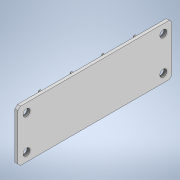
# Autodesk Inventor part: Halterung Gläser1,0
Saved by Autodesk Inventor 2021.3 (Build 253353000, 353)
## iProperties
Created: 2021-10-11
Part Number: Halterung Gläser1,0
Material: Generisch
Document SubType Name: Modeling
Designer: bhelg
Density: 1 g/cm^3
Appearance: Vorgabe
Author: bhelg
Autodesk Inventor part; units mm, degrees
ref_plane "YZ Plane" through (0, 0, 0) normal (1, 0, 0) x (0, 1, 0)
ref_plane "XZ Plane" through (0, 0, 0) normal (0, 1, 0) x (-1, 0, 0)
ref_plane "XY Plane" through (0, 0, 0) normal (0, 0, 1) x (1, 0, 0)
sketch "Skizze1" plane through (0, 0, 0) normal (0, 1, 0) x (-1, 0, 0)
  line L0 (10.8901, 21.3821) -> (14.3901, 21.3821)
  line L1 (14.3901, 21.3821) -> (14.3901, -158.6179)
  line L2 (14.3901, -158.6179) -> (10.8901, -158.6179)
  line L3 (10.8901, -158.6179) -> (10.8901, 21.3821)
  dimension "d0" = 180
  dimension "d1" = 3.5
  constraints: 8 end point, 3 perpendicular, 1 horizontal
  measures "d0" distance of L0.end L1.end
  measures "d1" distance of L0.start L0.end
extrude "Extrusion1" add sketch "Skizze1" along normal blind 60
sketch "Skizze2" plane through (-14.3901, 0, -158.6179) normal (-1, 0, 0) x (0, 0, 1)
  line L0 (0, 0) -> (180, 0) projected
  circle A0 centre (33, 16.5) radius 8.3 construction
  circle A1 centre (33, 43.5) radius 8.3 construction
  circle A2 centre (90, 30) radius 72.5 construction
  line L1 (0, 0) -> (0, 60) projected
  line L2 (0, 60) -> (180, 60) projected
  circle A3 centre (71, 16.5) radius 8.3 construction
  circle A4 centre (109, 16.5) radius 8.3 construction
  circle A5 centre (147, 16.5) radius 8.3 construction
  circle A6 centre (72.7786, 43.5) radius 8.3 construction
  circle A7 centre (109.0755, 43.5) radius 8.3 construction
  circle A8 centre (144.3092, 43.5) radius 8.3 construction
  circle A9 centre (33, 16.5) radius 9.8
  circle A10 centre (23.2, 16.5) radius 1.5
  circle A11 centre (33, 26.3) radius 1.5
  circle A12 centre (42.8, 16.5) radius 1.5
  circle A13 centre (33, 6.7) radius 1.5
  circle A14 centre (33, 43.5) radius 9.8
  circle A15 centre (23.2, 43.5) radius 1.5
  circle A16 centre (33, 53.3) radius 1.5
  circle A17 centre (42.8, 43.5) radius 1.5
  circle A18 centre (33, 33.7) radius 1.5
  point P0 (158.6179, 0)
  dimension "d38" = 16.6
  dimension "d39" = 16.6
  dimension "d42" = 145
  dimension "d43" = 90
  dimension "d44" = 30
  dimension "d50" = 33
  dimension "d51" = 33
  dimension "d52" = 16.5
  dimension "d53" = 16.5
  dimension "d63" = 16.6
  dimension "d64" = 16.6
  dimension "d65" = 16.6
  dimension "d66" = 16.6
  dimension "d67" = 16.6
  dimension "d68" = 16.6
  dimension "d69" = 38
  dimension "d70" = 38
  dimension "d71" = 38
  dimension "d98" = 19.6
  dimension "d99" = 3
  dimension "d100" = 3
  dimension "d101" = 3
  dimension "d102" = 3
  dimension "d103" = 19.6
  dimension "d104" = 3
  dimension "d105" = 3
  dimension "d106" = 3
  dimension "d107" = 3
  constraints: 19 centre point, 8 point on circle, 2 coincident
  measures "d38" diameter of A0
  measures "d39" diameter of A1
  measures "d42" diameter of A2
  measures "d43" horizontal distance of A2.centre L0.start
  measures "d44" vertical distance of L0.start A2.centre
  measures "d50" distance from line of L1 A0.centre
  measures "d51" distance from line of L1 A1.centre
  measures "d52" distance from line of L0 A0.centre
  measures "d53" distance from line of L2 A1.centre
  measures "d63" diameter of A3
  measures "d64" diameter of A4
  measures "d65" diameter of A5
  measures "d66" diameter of A6
  measures "d67" diameter of A7
  measures "d68" diameter of A8
  measures "d69" distance of A3.centre A0.centre
  measures "d70" distance of A4.centre A3.centre
  measures "d71" distance of A4.centre A5.centre
  measures "d98" diameter of A9
  measures "d99" diameter of A10
  measures "d100" diameter of A11
  measures "d101" diameter of A12
  measures "d102" diameter of A13
  measures "d103" diameter of A14
  measures "d104" diameter of A15
  measures "d105" diameter of A16
  measures "d106" diameter of A17
  measures "d107" diameter of A18
sketch "Skizze3" plane through (-14.3901, 0, -158.6179) normal (-1, 0, 0) x (0, 0, 1)
  line L0 (0, 0) -> (180, 0) projected
  line L1 (0, 60) -> (180, 60) projected
  line L2 (180, 0) -> (180, 60) projected
  line L3 (0, 0) -> (0, 60) projected
  line L4 (10, 10) -> (10, 50)
  point P0 (170, 10)
  point P1 (170, 50)
  dimension "d83" = 40
  dimension "d84" = 40
  dimension "d85" = 10
  dimension "d86" = 10
  dimension "d87" = 10
  dimension "d88" = 10
  dimension "d89" = 10
  dimension "d90" = 10
  dimension "d152" = 160
  constraints: 2 end point, 1 vertical
  measures "d83" distance of L4.end L4.start
  measures "d84" distance of point (170, 50) point (170, 10)
  measures "d85" distance from line of L0 point (170, 10)
  measures "d86" distance from line of L1 point (170, 50)
  measures "d87" distance from line of L0 L4.start
  measures "d88" distance from line of L1 L4.end
  measures "d89" distance from line of L2 point (170, 10)
  measures "d90" distance from line of L3 L4.start
  measures "d152" distance of point (170, 10) L4.start
hole "Bohrung1" at (-14.3901, 10, -148.6179) at (-14.3901, 50, -148.6179) at (-14.3901, 10, 11.3821) at (-14.3901, 50, 11.3821) direction (1, 0, 0) diameter 8.2 end through all
extrude "Extrusion3" add sketch "Skizze2" along normal blind 8 contours A9 A12 | A9 A12 | A11 A9 | A9 A11 | A13 A9 | A9 A13 | A10 A9 | A9 A10 | A14 A17 | A14 A17 | A16 A14 | A14 A16 | A18 A14 | A14 A18 | A15 A14 | A14 A15
pattern_linear "Rechteckige Anordnung2" count 4 spacing 37 along (0, 0, 1) of "Extrusion3"
fillet "Rundung1" radius 1 32 edges at (-22.3901, 6.7, -127.1179) (-22.3901, 16.5, -136.9179) (-22.3901, 16.5, -117.3179) (-22.3901, 26.3, -127.1179) (-22.3901, 33.7, -127.1179) (-22.3901, 43.5, -136.9179) (-22.3901, 43.5, -117.3179) (-22.3901, 53.3, -127.1179) (-22.3901, 16.5, -99.9179) (-22.3901, 6.7, -90.1179) (-22.3901, 26.3, -90.1179) (-22.3901, 33.7, -90.1179) (-22.3901, 43.5, -99.9179) (-22.3901, 16.5, -80.3179) (-22.3901, 53.3, -90.1179) (-22.3901, 43.5, -80.3179) (-22.3901, 43.5, -62.9179) (-22.3901, 33.7, -53.1179) (-22.3901, 26.3, -53.1179) (-22.3901, 16.5, -62.9179) (-22.3901, 6.7, -53.1179) (-22.3901, 16.5, -43.3179) (-22.3901, 16.5, -25.9179) (-22.3901, 6.7, -16.1179) (-22.3901, 16.5, -6.3179) (-22.3901, 26.3, -16.1179) (-22.3901, 33.7, -16.1179) (-22.3901, 43.5, -25.9179) (-22.3901, 43.5, -43.3179) (-22.3901, 53.3, -53.1179) (-22.3901, 53.3, -16.1179) (-22.3901, 43.5, -6.3179)
sketch "Skizze4" plane through (-14.3901, 0, -158.6179) normal (-1, 0, 0) x (0, 0, 1)
  line L0 (0, 0) -> (180, 0)
  circle A0 centre (33, 16.5) radius 8.3 construction
  circle A1 centre (33, 43.5) radius 8.3 construction
  circle A2 centre (90, 30) radius 72.5 construction
  line L1 (0, 0) -> (0, 60)
  line L2 (0, 60) -> (180, 60)
  circle A3 centre (71, 16.5) radius 8.3 construction
  circle A4 centre (109, 16.5) radius 8.3 construction
  circle A5 centre (147, 16.5) radius 8.3 construction
  circle A6 centre (72.7786, 43.5) radius 8.3 construction
  circle A7 centre (109.0755, 43.5) radius 8.3 construction
  circle A8 centre (144.3092, 43.5) radius 8.3 construction
  circle A9 centre (33, 16.5) radius 9.8
  circle A10 centre (23.2, 16.5) radius 1.5
  circle A11 centre (33, 26.3) radius 1.5
  circle A12 centre (42.8, 16.5) radius 1.5
  circle A13 centre (33, 6.7) radius 1.5
  circle A14 centre (33, 43.5) radius 9.8
  circle A15 centre (23.2, 43.5) radius 1.5
  circle A16 centre (33, 53.3) radius 1.5
  circle A17 centre (42.8, 43.5) radius 1.5
  circle A18 centre (33, 33.7) radius 1.5
  circle A19 centre (33, 16.5) radius 10.3
  circle A20 centre (33, 43.5) radius 10.3
  point P0 (158.6179, 0)
  point P1 (158.6179, 0)
  point P2 (31.5538, 53.698)
  point P3 (22.802, 44.9462)
  point P4 (23.3148, 44.9956)
  point P5 (31.5044, 53.1852)
  point P6 (22.802, 42.0538)
  point P7 (31.5538, 33.302)
  point P8 (31.5044, 33.8148)
  point P9 (23.3148, 42.0044)
  point P10 (34.4462, 33.302)
  point P11 (43.198, 42.0538)
  point P12 (42.6852, 42.0044)
  point P13 (34.4956, 33.8148)
  point P14 (43.198, 44.9462)
  point P15 (34.4462, 53.698)
  point P16 (34.4956, 53.1852)
  point P17 (42.6852, 44.9956)
  point P18 (31.5538, 26.698)
  point P19 (22.802, 17.9462)
  point P20 (23.3148, 17.9956)
  point P21 (31.5044, 26.1852)
  point P22 (22.802, 15.0538)
  point P23 (31.5538, 6.302)
  point P24 (31.5044, 6.8148)
  point P25 (23.3148, 15.0044)
  point P26 (43.198, 17.9462)
  point P27 (34.4462, 26.698)
  point P28 (34.4956, 26.1852)
  point P29 (42.6852, 17.9956)
  point P30 (34.4462, 6.302)
  point P31 (43.198, 15.0538)
  point P32 (42.6852, 15.0044)
  point P33 (34.4956, 6.8148)
  dimension "d114" = 16.6
  dimension "d115" = 16.6
  dimension "d116" = 145
  dimension "d117" = 90
  dimension "d118" = 30
  dimension "d119" = 33
  dimension "d120" = 33
  dimension "d121" = 16.5
  dimension "d122" = 16.5
  dimension "d123" = 16.6
  dimension "d124" = 16.6
  dimension "d125" = 16.6
  dimension "d126" = 16.6
  dimension "d127" = 16.6
  dimension "d128" = 16.6
  dimension "d129" = 38
  dimension "d130" = 38
  dimension "d131" = 38
  dimension "d132" = 19.6
  dimension "d133" = 3
  dimension "d134" = 3
  dimension "d135" = 3
  dimension "d136" = 3
  dimension "d137" = 19.6
  dimension "d138" = 3
  dimension "d139" = 3
  dimension "d140" = 3
  dimension "d141" = 3
  dimension "d142" = 20.6
  dimension "d143" = 20.6
  constraints: 21 centre point, 8 point on circle, 6 end point, 4 coincident
  measures "d114" diameter of A0
  measures "d115" diameter of A1
  measures "d116" diameter of A2
  measures "d117" horizontal distance of A2.centre L0.start
  measures "d118" vertical distance of L0.start A2.centre
  measures "d119" distance from line of L1 A0.centre
  measures "d120" distance from line of L1 A1.centre
  measures "d121" distance from line of L0 A0.centre
  measures "d122" distance from line of L2 A1.centre
  measures "d123" diameter of A3
  measures "d124" diameter of A4
  measures "d125" diameter of A5
  measures "d126" diameter of A6
  measures "d127" diameter of A7
  measures "d128" diameter of A8
  measures "d129" distance of A3.centre A0.centre
  measures "d130" distance of A4.centre A3.centre
  measures "d131" distance of A4.centre A5.centre
  measures "d132" diameter of A9
  measures "d133" diameter of A10
  measures "d134" diameter of A11
  measures "d135" diameter of A12
  measures "d136" diameter of A13
  measures "d137" diameter of A14
  measures "d138" diameter of A15
  measures "d139" diameter of A16
  measures "d140" diameter of A17
  measures "d141" diameter of A18
  measures "d142" diameter of A19
  measures "d143" diameter of A20
extrude "Extrusion4" cut sketch "Skizze4" against normal blind 0.5 contours A9 A11 A19 A12 | A12 A19 A13 A9 | A9 A10 A19 A11 | A13 A19 A10 A9 | A14 A16 A20 A17 | A17 A20 A18 A14 | A14 A15 A20 A16 | A18 A20 A15 A14
pattern_linear "Rechteckige Anordnung3" count 4 spacing 37 along (0, 0, 1) of "Extrusion4"
chamfer "Fase1" distance 3 angle 45 4 edges at (-12.6401, 60, 21.3821) (-12.6401, 0, 21.3821) (-12.6401, 0, -158.6179) (-12.6401, 60, -158.6179)
